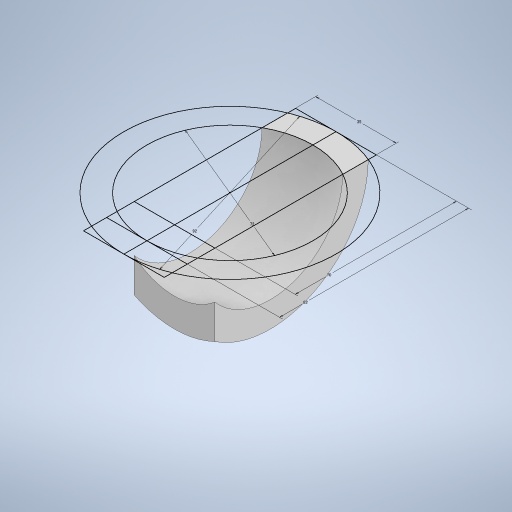
# Autodesk Inventor part: tail trying like shit
Saved by Autodesk Inventor 2023 (Build 270158000, 158)
## iProperties
Created: 2022-10-30
Part Number: tail trying like shit
Material: 一般
Document SubType Name: Modeling
Designer: RM206user
Density: 1 g/cm^3
Appearance: 既定
Author: RM206user
Autodesk Inventor part; units mm, degrees
ref_plane "YZ Plane" through (0, 0, 0) normal (1, 0, 0) x (0, 1, 0)
ref_plane "XZ Plane" through (0, 0, 0) normal (0, 1, 0) x (-1, 0, 0)
ref_plane "XY Plane" through (0, 0, 0) normal (0, 0, 1) x (1, 0, 0)
sketch "スケッチ1" plane through (0, 0, 0) normal (0, 1, 0) x (-1, 0, 0)
  circle A0 centre (0, 0) radius 36
  circle A1 centre (0, 0) radius 46
  line L0 (0, -46) -> (0, 46)
  line L1 (17.5, -46) -> (-17.5, -46)
  line L2 (-17.5, -46) -> (-17.5, 46)
  line L3 (-17.5, 46) -> (17.5, 46)
  line L4 (17.5, 46) -> (17.5, -46)
  line L5 (17.5, 24) -> (-17.5, 24)
  line L6 (17.5, 36) -> (-17.5, 36)
  point P0 (0, 36)
  point P1 (0, -36)
  point P2 (-17.5, 42.5412)
  point P3 (-17.5, -42.5412)
  point P4 (17.5, -42.5412)
  point P5 (17.5, 42.5412)
  dimension "d0" = 72
  dimension "d1" = 92
  dimension "d4" = 35
  dimension "d7" = 70
  dimension "d10" = 82
  constraints: 14 end point, 4 point on line, 3 horizontal, 2 centre point, 2 coincident, 2 parallel, 2 point on circle, 2 tangent, 1 line through centre, 1 perpendicular, 1 vertical, 1 other
  measures "d0" diameter of A0
  measures "d1" diameter of A1
  measures "d4" distance between parallel lines of L2 L4
  measures "d7" distance between parallel lines of L5 L1
  measures "d10" distance between parallel lines of L6 L1
revolve "回転1" add sketch "スケッチ1" angle 180 about axis through (0, 0, -46) along (0, 0, 1) contours A0 L4 | A0 L4 A1 | L4 L5 L0 A0 | A0 L6 L4 | L4 A1 L0 A0 | A0 L0 L5 L4 | L0 A1 L4 L6
revolve "回転2" cut sketch "スケッチ1" angle 180 about axis through (0, 0, -46) along (0, 0, 1) contours A0 L4 | L4 L5 L0 A0 | A0 L0 L5 L4
extrude "押し出し1" cut sketch "スケッチ1" against normal blind 150 contours A0 L4 | A0 L4 A1 | L2 A0 | A0 L2 A1
extrude "押し出し2" cut sketch "スケッチ1" against normal blind 150 contours L4 L5 L0 A0 | A0 L6 L4 | L0 L5 L2 A0 | L6 L2 A1 L0 | L0 A1 L4 L6 | A0 L2 L6 picked at (9.8173, 27.3194) picked at (-9.8173, 27.3194)
